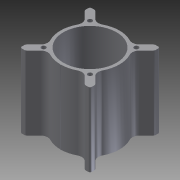
# Autodesk Inventor part: X95_100mm
Saved by Autodesk Inventor 2012 SP2 (Build 160219200, 219)
## iProperties
Created: 2012-04-18
Part Number: X95_100mm
Document SubType Name: Modeling
Designer: Fabian
Density: 1 g/cm^3
Material: Default
Author: Fabian
Autodesk Inventor part; units mm, degrees
ref_plane "YZ Plane" through (0, 0, 0) normal (1, 0, 0) x (0, 1, 0)
ref_plane "XZ Plane" through (0, 0, 0) normal (0, 1, 0) x (-1, 0, 0)
ref_plane "XY Plane" through (0, 0, 0) normal (0, 0, 1) x (1, 0, 0)
sketch "Sketch1" plane through (0, 0, 0) normal (0, 0, 1) x (1, 0, 0)
  arc A0 (11.6951, -1.7956) -> (0, 0) centre (4.624, -8.8667) ccw
  line L0 (11.6951, -1.7956) -> (21.2005, -11.301)
  arc A1 (21.2005, -11.301) -> (22.9683, -12.0332) centre (22.9683, -9.5332) ccw
  line L1 (22.9683, -12.0332) -> (26.5038, -12.0332)
  arc A2 (26.5038, -12.0332) -> (29.0038, -9.5332) centre (26.5038, -9.5332) ccw
  line L2 (29.0038, -9.5332) -> (29.0038, -5.9977)
  arc A3 (29.0038, -5.9977) -> (28.2716, -4.2299) centre (26.5038, -5.9977) ccw
  line L3 (28.2716, -4.2299) -> (18.7662, 5.2754)
  arc A4 (16.9706, 16.9706) -> (18.7662, 5.2754) centre (25.8373, 12.3465) ccw
  arc A5 (16.9706, 16.9706) -> (16.9706, 53.963) centre (-18.4962, 35.4668) ccw
  arc A6 (18.7662, 65.6581) -> (16.9706, 53.963) centre (25.8373, 58.587) ccw
  line L4 (18.7662, 65.6581) -> (28.2716, 75.1635)
  arc A7 (28.2716, 75.1635) -> (29.0038, 76.9312) centre (26.5038, 76.9312) ccw
  line L5 (29.0038, 76.9312) -> (29.0038, 80.4668)
  arc A8 (29.0038, 80.4668) -> (26.5038, 82.9668) centre (26.5038, 80.4668) ccw
  line L6 (26.5038, 82.9668) -> (22.9683, 82.9668)
  arc A9 (22.9683, 82.9668) -> (21.2005, 82.2345) centre (22.9683, 80.4668) ccw
  line L7 (21.2005, 82.2345) -> (11.6951, 72.7291)
  arc A10 (0, 70.9335) -> (11.6951, 72.7291) centre (4.624, 79.8002) ccw
  arc A11 (0, 70.9335) -> (-36.9924, 70.9335) centre (-18.4962, 35.4668) ccw
  arc A12 (-48.6875, 72.7291) -> (-36.9924, 70.9335) centre (-41.6164, 79.8002) ccw
  line L8 (-48.6875, 72.7291) -> (-58.1929, 82.2345)
  arc A13 (-58.1929, 82.2345) -> (-59.9607, 82.9668) centre (-59.9607, 80.4668) ccw
  line L9 (-59.9607, 82.9668) -> (-63.4962, 82.9668)
  arc A14 (-63.4962, 82.9668) -> (-65.9962, 80.4668) centre (-63.4962, 80.4668) ccw
  line L10 (-65.9962, 80.4668) -> (-65.9962, 76.9312)
  arc A15 (-65.9962, 76.9312) -> (-65.264, 75.1635) centre (-63.4962, 76.9312) ccw
  line L11 (-65.264, 75.1635) -> (-55.7586, 65.6581)
  arc A16 (-53.9629, 53.963) -> (-55.7586, 65.6581) centre (-62.8296, 58.587) ccw
  arc A17 (-53.9629, 53.963) -> (-53.963, 16.9706) centre (-18.4962, 35.4668) ccw
  arc A18 (-55.7586, 5.2754) -> (-53.963, 16.9706) centre (-62.8296, 12.3465) ccw
  line L12 (-55.7586, 5.2754) -> (-65.264, -4.2299)
  arc A19 (-65.264, -4.2299) -> (-65.9962, -5.9977) centre (-63.4962, -5.9977) ccw
  line L13 (-65.9962, -5.9977) -> (-65.9962, -9.5332)
  arc A20 (-65.9962, -9.5332) -> (-63.4962, -12.0332) centre (-63.4962, -9.5332) ccw
  line L14 (-63.4962, -12.0332) -> (-59.9607, -12.0332)
  arc A21 (-59.9607, -12.0332) -> (-58.1929, -11.301) centre (-59.9607, -9.5332) ccw
  line L15 (-58.1929, -11.301) -> (-48.6875, -1.7956)
  arc A22 (-36.9924, 0) -> (-48.6875, -1.7956) centre (-41.6164, -8.8667) ccw
  arc A23 (-36.9924, 0) -> (-18.9962, -4.5301) centre (-18.4962, 35.4668) ccw
  arc A24 (-18.9962, -4.5301) -> (-17.9962, -4.5301) centre (-18.4962, -4.5332) ccw
  arc A25 (-17.9962, -4.5301) -> (0, 0) centre (-18.4962, 35.4668) ccw
  circle A26 centre (-49.9962, 3.9668) radius 3
  circle A27 centre (-49.9962, 66.9668) radius 3
  circle A28 centre (13.0038, 3.9668) radius 3
  circle A29 centre (13.0038, 66.9668) radius 3
  circle A30 centre (-18.4962, 35.4668) radius 36
extrude "Extrusion1" add sketch "Sketch1" along normal blind 400
sketch "Sketch2" plane through (0, 0, 400) normal (0, 0, 1) x (1, 0, 0)
  circle A0 centre (-18.4962, 35.4668) radius 36 projected
  circle A1 centre (13.0038, 66.9668) radius 3 projected
  circle A2 centre (13.0038, 3.9668) radius 3 projected
  circle A3 centre (-49.9962, 66.9668) radius 3 projected
  circle A4 centre (-49.9962, 3.9668) radius 3 projected
  arc A5 (-17.9962, -4.5301) -> (0, 0) centre (-18.4962, 35.4668) ccw projected
  arc A6 (11.6951, -1.7956) -> (0, 0) centre (4.624, -8.8667) ccw projected
  line L0 (21.2005, -11.301) -> (11.6951, -1.7956) projected
  arc A7 (21.2005, -11.301) -> (22.9683, -12.0332) centre (22.9683, -9.5332) ccw projected
  line L1 (26.5038, -12.0332) -> (22.9683, -12.0332) projected
  arc A8 (26.5038, -12.0332) -> (29.0038, -9.5332) centre (26.5038, -9.5332) ccw projected
  line L2 (29.0038, -5.9977) -> (29.0038, -9.5332) projected
  arc A9 (29.0038, -5.9977) -> (28.2716, -4.2299) centre (26.5038, -5.9977) ccw projected
  line L3 (18.7662, 5.2754) -> (28.2716, -4.2299) projected
  arc A10 (16.9706, 16.9706) -> (18.7662, 5.2754) centre (25.8373, 12.3465) ccw projected
  arc A11 (16.9706, 16.9706) -> (16.9706, 53.963) centre (-18.4962, 35.4668) ccw projected
  arc A12 (18.7662, 65.6581) -> (16.9706, 53.963) centre (25.8373, 58.587) ccw projected
  line L4 (28.2716, 75.1635) -> (18.7662, 65.6581) projected
  arc A13 (28.2716, 75.1635) -> (29.0038, 76.9312) centre (26.5038, 76.9312) ccw projected
  line L5 (29.0038, 80.4668) -> (29.0038, 76.9312) projected
  arc A14 (29.0038, 80.4668) -> (26.5038, 82.9668) centre (26.5038, 80.4668) ccw projected
  line L6 (22.9683, 82.9668) -> (26.5038, 82.9668) projected
  arc A15 (22.9683, 82.9668) -> (21.2005, 82.2345) centre (22.9683, 80.4668) ccw projected
  line L7 (11.6951, 72.7291) -> (21.2005, 82.2345) projected
  arc A16 (0, 70.9335) -> (11.6951, 72.7291) centre (4.624, 79.8002) ccw projected
  arc A17 (0, 70.9335) -> (-36.9924, 70.9335) centre (-18.4962, 35.4668) ccw projected
  arc A18 (-48.6875, 72.7291) -> (-36.9924, 70.9335) centre (-41.6164, 79.8002) ccw projected
  line L8 (-58.1929, 82.2345) -> (-48.6875, 72.7291) projected
  arc A19 (-58.1929, 82.2345) -> (-59.9607, 82.9668) centre (-59.9607, 80.4668) ccw projected
  line L9 (-63.4962, 82.9668) -> (-59.9607, 82.9668) projected
  arc A20 (-63.4962, 82.9668) -> (-65.9962, 80.4668) centre (-63.4962, 80.4668) ccw projected
  line L10 (-65.9962, 76.9312) -> (-65.9962, 80.4668) projected
  arc A21 (-65.9962, 76.9312) -> (-65.264, 75.1635) centre (-63.4962, 76.9312) ccw projected
  line L11 (-55.7586, 65.6581) -> (-65.264, 75.1635) projected
  arc A22 (-53.9629, 53.963) -> (-55.7586, 65.6581) centre (-62.8296, 58.587) ccw projected
  arc A23 (-53.9629, 53.963) -> (-53.963, 16.9706) centre (-18.4962, 35.4668) ccw projected
  arc A24 (-55.7586, 5.2754) -> (-53.963, 16.9706) centre (-62.8296, 12.3465) ccw projected
  line L12 (-65.264, -4.2299) -> (-55.7586, 5.2754) projected
  arc A25 (-65.264, -4.2299) -> (-65.9962, -5.9977) centre (-63.4962, -5.9977) ccw projected
  line L13 (-65.9962, -9.5332) -> (-65.9962, -5.9977) projected
  arc A26 (-65.9962, -9.5332) -> (-63.4962, -12.0332) centre (-63.4962, -9.5332) ccw projected
  line L14 (-59.9607, -12.0332) -> (-63.4962, -12.0332) projected
  arc A27 (-59.9607, -12.0332) -> (-58.1929, -11.301) centre (-59.9607, -9.5332) ccw projected
  line L15 (-48.6875, -1.7956) -> (-58.1929, -11.301) projected
  arc A28 (-36.9924, 0) -> (-48.6875, -1.7956) centre (-41.6164, -8.8667) ccw projected
  arc A29 (-36.9924, 0) -> (-18.9962, -4.5301) centre (-18.4962, 35.4668) ccw projected
  arc A30 (-18.9962, -4.5301) -> (-17.9962, -4.5301) centre (-18.4962, -4.5332) ccw projected
extrude "Extrusion2" cut sketch "Sketch2" against normal blind 250
sketch "Sketch3" plane through (-63.4962, -12.0332, 0) normal (0, -1, 0) x (1, 0, 0)
  line L0 (0, 0) -> (0, 150) projected
  line L1 (-3.0046, 150) -> (99.6718, 150)
  line L2 (99.6718, 150) -> (99.6718, 100)
  line L3 (99.6718, 100) -> (-3.0046, 100)
  line L4 (-3.0046, 100) -> (-3.0046, 150)
  point P0 (63.4962, 0)
  dimension "d4" = 50
  dimension "d5" = 102.6763
  dimension "d6" = 3.0046
  constraints: 8 end point, 2 parallel, 1 horizontal, 1 perpendicular
  measures "d4" distance of L1.end L2.end
  measures "d5" distance of L1.start L1.end
  measures "d6" distance between parallel lines of L4 L0
extrude "Extrusion3" cut sketch "Sketch3" against normal blind 95
body "Solid1"
